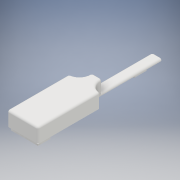
# Autodesk Inventor part: POVlid
Saved by Autodesk Inventor 2017 SP1 (Build 210196100, 196)
## iProperties
Created: 2016-11-21
Part Number: POVlid
Material: ABS Plastic
Document SubType Name: Modeling
Designer: bzs3334
Density: 1.06 g/cm^3
Appearance: Smooth - White
Mass: 5.67284 g
Surface Area: 63.4072 cm^2
Volume: 5.35174 cm^3
Author: bzs3334
Autodesk Inventor part; units mm, degrees
ref_plane "YZ Plane" through (0, 0, 0) normal (1, 0, 0) x (0, 1, 0)
ref_plane "XZ Plane" through (0, 0, 0) normal (0, 1, 0) x (-1, 0, 0)
ref_plane "XY Plane" through (0, 0, 0) normal (0, 0, 1) x (1, 0, 0)
sketch "Sketch3" plane through (0, 0, 0) normal (0, 0, 1) x (1, 0, 0)
  arc A0 (-3, 115) -> (-5, 113) centre (-3, 113) ccw
  line L0 (-5, 113) -> (-5, 54.5)
  arc A1 (-13.3333, 44.6399) -> (-5, 54.5) centre (-15, 54.5) ccw
  arc A2 (-13.3333, 44.6399) -> (-15, 42.6678) centre (-13, 42.6678) ccw
  line L1 (-15, 42.6678) -> (-15, -13.5)
  arc A3 (-15, -13.5) -> (-13, -15.5) centre (-13, -13.5) ccw
  line L2 (-13, -15.5) -> (13, -15.5)
  arc A4 (13, -15.5) -> (15, -13.5) centre (13, -13.5) ccw
  line L3 (15, -13.5) -> (15, 42.6678)
  arc A5 (15, 42.6678) -> (13.3333, 44.6399) centre (13, 42.6678) ccw
  arc A6 (5, 54.5) -> (13.3333, 44.6399) centre (15, 54.5) ccw
  line L4 (5, 54.5) -> (5, 113)
  arc A7 (5, 113) -> (3, 115) centre (3, 113) ccw
  line L5 (3, 115) -> (-3, 115)
  line L6 (13, -2.8322) -> (13.5, -2.8322)
  line L7 (13.5, -2.8322) -> (13.5, -3.5)
  line L8 (13.5, -3.5) -> (-13.5, -3.5)
  line L9 (-13.5, -3.5) -> (-13.5, 7.1678)
  line L10 (-13.5, 7.1678) -> (-13, 7.1678)
  arc A8 (-13, 7.1678) -> (-3, 19) centre (-15, 19) ccw
  line L11 (-3, 19) -> (-3, 110.7727)
  line L12 (3, 100.7727) -> (3, 9)
  arc A9 (3, 9) -> (13, -2.8322) centre (15, 9) ccw
  line L13 (-13.5, -3.5) -> (13.5, -3.5)
  line L14 (13.5, -3.5) -> (13.5, -13.5)
  line L15 (13.5, -13.5) -> (-13.5, -13.5)
  line L16 (-13.5, -13.5) -> (-13.5, -3.5)
  line L17 (13.5, -3.5) -> (-13.5, -3.5)
  line L18 (-13.5, -3.5) -> (-13.5, -1.5)
  line L19 (-13.5, -1.5) -> (13.5, -1.5)
  line L20 (13.5, -1.5) -> (13.5, -3.5)
  line L21 (13.5, -1.5) -> (13, -1.5)
  line L22 (13, -1.5) -> (13, -3.5)
  line L23 (13, -3.5) -> (13.5, -3.5)
  line L24 (13.5, -3.5) -> (13.5, -1.5)
  line L25 (-13.5, -3.5) -> (-13, -3.5)
  line L26 (-13, -3.5) -> (-13, -1.5)
  line L27 (-13, -1.5) -> (-13.5, -1.5)
  line L28 (-13.5, -1.5) -> (-13.5, -3.5)
  line L29 (3, 113) -> (-3, 113)
  line L30 (-3, 113) -> (-3, 100)
  line L31 (-3, 100) -> (3, 100)
  line L32 (3, 100) -> (3, 113)
  line L33 (3, 100) -> (-3, 100)
  line L34 (-3, 100) -> (-3, 102)
  line L35 (-3, 102) -> (3, 102)
  line L36 (3, 102) -> (3, 100)
  line L37 (3, 102) -> (2.5, 102)
  line L38 (2.5, 102) -> (2.5, 100)
  line L39 (2.5, 100) -> (3, 100)
  line L40 (3, 100) -> (3, 102)
  line L41 (-3, 102) -> (-2.5, 102)
  line L42 (-2.5, 102) -> (-2.5, 100)
  line L43 (-2.5, 100) -> (-3, 100)
  line L44 (-3, 100) -> (-3, 102)
  line L45 (-2.5, 102) -> (2.5, 102)
  line L46 (2.5, 102) -> (2.5, 100)
  line L47 (2.5, 100) -> (-2.5, 100)
  line L48 (-2.5, 100) -> (-2.5, 102)
  line L49 (2.5, 102) -> (3, 102)
  line L50 (3, 102) -> (3, 100)
  line L51 (3, 100) -> (2.5, 100)
  line L52 (2.5, 100) -> (2.5, 102)
  line L53 (-5, 54.5) -> (5, 54.5)
  line L54 (13, 42.6678) -> (-13, 42.6678)
  point P0 (0, 0)
  point P1 (0, 0)
  dimension "d21" = 2
  dimension "d28" = 0.5
  dimension "d29" = 0.5
  dimension "d34" = 13
  dimension "d35" = 2
  dimension "d36" = 0.5
  dimension "d37" = 0.5
  dimension "d46" = 10
  dimension "d47" = 2
  dimension "d49" = 45.5
  constraints: 110 end point, 20 parallel, 20 point on circle, 11 horizontal, 11 perpendicular, 10 centre point, 7 point on line
  measures "d21" distance of L17.end L18.end
  measures "d28" distance of L23.end L22.end
  measures "d29" distance of L27.end L26.end
  measures "d34" distance of L30.end L29.end
  measures "d35" distance of L33.end L34.end
  measures "d36" distance of L39.end L38.end
  measures "d37" distance of L42.end L43.end
  measures "d46" distance between parallel lines of L15 L8
  measures "d47" distance between parallel lines of L15 L2
  measures "d49" distance between parallel lines of L47 L53
extrude "Extrusion2" add sketch "Sketch3" along normal blind 2
extrude "Extrusion3" add sketch "Sketch3" against normal blind 3.5 contours L19 L22 A9 | A9 L22 L8 L26 L19 | L19 L26 L8 L9 | L22 L19 L20 L6 | L6 L7 L8 L22
sketch "Sketch4" plane through (-13.5, -3.5, 0) normal (0, -1, 0) x (1, 0, 0)
  line L0 (0, 0) -> (27, 0) projected
  line L1 (0, 0) -> (0, -3.5) projected
  line L2 (27, -3.5) -> (0, -3.5) projected
  line L3 (27, 0) -> (27, -3.5) projected
  line L4 (0, -3.5) -> (27, -3.5) projected
  line L5 (0, 0) -> (0, -3.5) projected
  line L6 (27, -3.5) -> (0, -3.5)
  line L7 (0, -3.5) -> (0, -2)
  line L8 (0, -2) -> (27, -2)
  line L9 (27, -2) -> (27, -3.5)
  point P0 (13.5, 0)
  dimension "d24" = 1.5
  constraints: 8 end point, 2 parallel, 1 horizontal, 1 perpendicular, 1 point on line
  measures "d24" distance of L6.end L7.end
extrude "Extrusion4" add sketch "Sketch4" along normal blind 10 contours L8 L3 L2 L1
extrude "Extrusion5" cut sketch "Sketch3" against normal through all contours L22 L19 L20 L6 | L6 L7 L8 L22
mirror "Mirror1" about plane through (0, 0, 0) normal (1, 0, 0) of "Extrusion5"
sketch "Sketch5" plane through (13.5, -13.5, -2) normal (1, 0, 0) x (0, 0, -1)
  line L0 (1.5, 10) -> (0, 10) projected
  line L1 (0, 10) -> (0, 0) projected
  line L2 (1.5, 0) -> (0, 0) projected
  line L3 (1.5, 10) -> (1.5, 0) projected
  point P0 (-2, 13.5)
extrude "Extrusion6" cut sketch "Sketch5" against normal up to surface (0.5 mm away)
mirror "Mirror2" about plane through (0, 0, 0) normal (1, 0, 0) of "Extrusion6"
extrude "Extrusion7" add sketch "Sketch3" against normal blind 3.5 contours L11 L35 L42 L31 | L42 L35 L38 L31 | L31 L38 L35 L32 L12
extrude "Extrusion8" cut sketch "Sketch3" against normal through all contours L31 L38 L35 L32 L12
mirror "Mirror3" about plane through (0, 0, 0) normal (1, 0, 0) of "Extrusion8"
sketch "Sketch6" plane through (2.5, 100, -3.5) normal (0, -1, 0) x (1, 0, 0)
  line L0 (-5, 0) -> (-5, 3.5) projected
  line L1 (0, 3.5) -> (-5, 3.5) projected
  line L2 (0, 3.5) -> (0, 0) projected
  line L3 (-5, 0) -> (0, 0) projected
  line L4 (-5, 0) -> (-5, 3.5) projected
  line L5 (0, 0) -> (-5, 0)
  line L6 (-5, 0) -> (-5, 1.5)
  line L7 (-5, 1.5) -> (0, 1.5)
  line L8 (0, 1.5) -> (0, 0)
  point P0 (-2.5, 3.5)
  dimension "d42" = 1.5
  constraints: 8 end point, 2 parallel, 1 horizontal, 1 perpendicular, 1 point on line
  measures "d42" distance of L5.end L6.end
extrude "Extrusion9" add sketch "Sketch6" along normal blind 10 contours L0 L7 L2 L3
sketch "Sketch7" plane through (0, 0, 0) normal (0, 0, -1) x (-1, 0, 0)
  line L0 (13, -1.5) -> (-13, -1.5) projected
  line L1 (-13, 42.6678) -> (-13, -13.5) projected
  arc A0 (3, 54.5) -> (13, 42.6678) centre (15, 54.5) ccw projected
  arc A1 (-13, 42.6678) -> (-3, 54.5) centre (-15, 54.5) ccw projected
  line L2 (2.5, 100) -> (-2.5, 100) projected
  line L3 (-2.5, 102) -> (-2.5, 100) projected
  line L4 (-2.5, 102) -> (2.5, 102) projected
  line L5 (2.5, 102) -> (2.5, 100) projected
  line L6 (13, -3.5) -> (-13, -3.5) projected
  line L7 (-13, -1.5) -> (-13, -3.5) projected
  line L8 (-13, -1.5) -> (13, -1.5) projected
  line L9 (13, -1.5) -> (13, -3.5) projected
  line L10 (13, -13.5) -> (13, 42.6678) projected
  line L11 (-13, -1.5) -> (13, -1.5) projected
  line L12 (-13, -1.5) -> (13, -1.5)
  line L13 (13, -1.5) -> (13, 42.6678)
  line L14 (13, 42.6678) -> (-13, 42.6678)
  line L15 (-13, 42.6678) -> (-13, -1.5)
  point P0 (0, 0)
  constraints: 8 end point, 2 parallel, 1 horizontal, 1 perpendicular
extrude "Extrusion10" cut sketch "Sketch7" against normal through all contours L0 L1 L14 L10
sketch "Sketch8" plane through (0, 0, 2) normal (0, 0, 1) x (1, 0, 0)
  line L0 (-13, -1.5) -> (-13, 42.6678) projected
  line L1 (-13, 42.6678) -> (13, 42.6678) projected
  line L2 (13, 42.6678) -> (13, -1.5) projected
  line L3 (13, -1.5) -> (-13, -1.5) projected
  arc A0 (-3, 115) -> (-5, 113) centre (-3, 113) ccw projected
  line L4 (-5, 113) -> (-5, 54.5) projected
  arc A1 (-13.3333, 44.6399) -> (-5, 54.5) centre (-15, 54.5) ccw projected
  arc A2 (-13.3333, 44.6399) -> (-15, 42.6678) centre (-13, 42.6678) ccw projected
  line L5 (-15, 42.6678) -> (-15, -13.5) projected
  arc A3 (-15, -13.5) -> (-13, -15.5) centre (-13, -13.5) ccw projected
  line L6 (-13, -15.5) -> (13, -15.5) projected
  arc A4 (13, -15.5) -> (15, -13.5) centre (13, -13.5) ccw projected
  line L7 (15, -13.5) -> (15, 42.6678) projected
  arc A5 (15, 42.6678) -> (13.3333, 44.6399) centre (13, 42.6678) ccw projected
  arc A6 (5, 54.5) -> (13.3333, 44.6399) centre (15, 54.5) ccw projected
  line L8 (5, 54.5) -> (5, 113) projected
  arc A7 (5, 113) -> (3, 115) centre (3, 113) ccw projected
  line L9 (3, 115) -> (-3, 115) projected
  line L10 (-3, 54.5) -> (3, 54.5)
  line L11 (13, 42.6678) -> (-13, 42.6678) projected
  line L12 (-3, 56.5) -> (-3, 113)
  line L13 (-3, 113) -> (3, 113)
  line L14 (3, 113) -> (3, 56.5)
  arc A8 (3, 54.5) -> (13, 42.6678) centre (15, 54.5) ccw
  line L15 (13, 42.6678) -> (13, -13.5)
  line L16 (13, -13.5) -> (-13, -13.5)
  line L17 (-13, -13.5) -> (-13, 42.6678)
  arc A9 (-13, 42.6678) -> (-3, 54.5) centre (-15, 54.5) ccw
  line L18 (-13, 42.6678) -> (13, 42.6678)
  line L19 (-3, 54.5) -> (3, 54.5)
  line L20 (-5, 56.5) -> (5, 56.5)
  line L21 (5, 54.5) -> (5, 113) projected
  line L22 (-5, 54.5) -> (-5, 56.5)
  line L23 (5, 56.5) -> (5, 54.5)
  line L24 (-3, 54.5) -> (3, 54.5)
  line L25 (-5, 56.5) -> (5, 56.5)
  point P0 (0, 0)
  dimension "d52" = 2
  dimension "d55" = 2
  dimension "d56" = 2
  constraints: 28 end point, 4 point on circle, 4 point on line, 3 perpendicular, 2 centre point, 2 horizontal, 2 parallel, 1 collinear, 4 other
  measures "d52" radial gap between concentric circles of A1 A9
  measures "d55" distance between parallel lines of L19 L20
  measures "d56" distance from line of L4 L10.start
extrude "Extrusion11" cut sketch "Sketch8" against normal through all contours A9 L10 A8 L1
extrude "Extrusion12" add sketch "Sketch8" along normal blind 10 contours L20 L8 A6 A5 L7 A4 L6 A3 L5 A2 A1 L4
sketch "Sketch9" plane through (0, 0, 12) normal (0, 0, 1) x (1, 0, 0)
  arc A0 (-13.3333, 44.6399) -> (-5, 54.5) centre (-15, 54.5) ccw projected
  arc A1 (-13.3333, 44.6399) -> (-15, 42.6678) centre (-13, 42.6678) ccw projected
  line L0 (-15, 42.6678) -> (-15, -13.5) projected
  arc A2 (-15, -13.5) -> (-13, -15.5) centre (-13, -13.5) ccw projected
  line L1 (-13, -15.5) -> (13, -15.5) projected
  arc A3 (13, -15.5) -> (15, -13.5) centre (13, -13.5) ccw projected
  line L2 (15, -13.5) -> (15, 42.6678) projected
  arc A4 (15, 42.6678) -> (13.3333, 44.6399) centre (13, 42.6678) ccw projected
  arc A5 (5, 54.5) -> (13.3333, 44.6399) centre (15, 54.5) ccw projected
  line L3 (5, 54.5) -> (5, 56.5) projected
  line L4 (5, 56.5) -> (-5, 56.5) projected
  line L5 (-5, 56.5) -> (-5, 54.5) projected
  line L6 (13, 42.6678) -> (13, -13.5) projected
  line L7 (13, -13.5) -> (-13, -13.5) projected
  line L8 (-13, -13.5) -> (-13, 42.6678) projected
  arc A6 (-13, 42.6678) -> (-3, 54.5) centre (-15, 54.5) ccw projected
  line L9 (-3, 54.5) -> (3, 54.5) projected
  arc A7 (3, 54.5) -> (13, 42.6678) centre (15, 54.5) ccw projected
  point P0 (0, 0)
extrude "Extrusion13" add sketch "Sketch9" along normal blind 2 contours A0 L5 L4 L3 A5 A4 L2 A3 L1 A2 L0 A1 | L6 L7 L8 A6 L9 A7
fillet "Fillet2" radius 2 11 edges at (14.4142, -14.9142, 14) (15, 14.5839, 14) (14.5275, 43.9588, 14) (7.3624, 48.045, 14) (5, 55.5, 14) (-14.4142, -14.9142, 14) (-15, 14.5839, 14) (-14.5275, 43.9588, 14) (-7.3624, 48.045, 14) (-5, 55.5, 14) (0, -15.5, 14)
sketch "Sketch10" plane through (-5, 56.5, 2) normal (0, 1, 0) x (1, 0, 0)
  arc A0 (0, -10) -> (2, -12) centre (2, -10) ccw projected
  line L0 (8, -12) -> (2, -12) projected
  arc A1 (8, -12) -> (10, -10) centre (8, -10) ccw projected
  line L1 (10, 0) -> (10, -10) projected
  line L2 (0, 0) -> (10, 0) projected
  line L3 (0, 0) -> (0, -10) projected
  line L4 (6.5, -6.5) -> (3.5, -6.5)
  line L5 (3.5, -6.5) -> (3.5, -1.5)
  line L6 (3.5, -1.5) -> (6.5, -1.5)
  line L7 (6.5, -1.5) -> (6.5, -6.5)
  point P0 (5, 2)
  dimension "d62" = 3
  dimension "d63" = 5
  dimension "d64" = 3.5
  dimension "d65" = 1.5
  constraints: 8 end point, 2 parallel, 1 horizontal, 1 perpendicular
  measures "d62" distance of L5.end L6.end
  measures "d63" distance of L4.end L5.end
  measures "d64" distance between parallel lines of L1 L7
  measures "d65" distance between parallel lines of L2 L6
extrude "Extrusion14" cut sketch "Sketch10" against normal blind 2 contours L4 L5 L6 L7
fillet "Fillet3" radius 2 10 edges at (4.4142, 114.4142, 2) (0, 115, 2) (-4.4142, 114.4142, 2) (-5, 84.75, 2) (5, 84.75, 2) (-4.4142, 56.5, 13.4142) (-5, 56.5, 7) (4.4142, 56.5, 13.4142) (5, 56.5, 7) (0, 56.5, 14)
body "Solid2"
